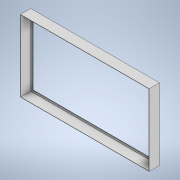
# Autodesk Inventor part: marco_ir
Saved by Autodesk Inventor 2021 (Build 250183000, 183)
## iProperties
Created: 2021-11-08
Part Number: marco_ir
Material: Genérico
Document SubType Name: Modeling
Designer: arthu
Density: 1 g/cm^3
Appearance: Valor por defecto
Author: arthu
Autodesk Inventor part; units mm, degrees
ref_plane "YZ Plane" through (0, 0, 0) normal (1, 0, 0) x (0, 1, 0)
ref_plane "XZ Plane" through (0, 0, 0) normal (0, 1, 0) x (-1, 0, 0)
ref_plane "XY Plane" through (0, 0, 0) normal (0, 0, 1) x (1, 0, 0)
sketch "Boceto1" plane through (0, 0, 0) normal (0, 0, 1) x (1, 0, 0)
  line L0 (260, -145) -> (-260, -145)
  line L1 (-260, -145) -> (-260, 145)
  line L2 (-260, 145) -> (260, 145)
  line L3 (260, 145) -> (260, -145)
  line L4 (260, -145) -> (-260, 145) construction
  line L5 (-260, -145) -> (260, 145) construction
  line L6 (250, -135) -> (-250, -135)
  line L7 (-250, -135) -> (-250, 135)
  line L8 (-250, 135) -> (250, 135)
  line L9 (250, 135) -> (250, -135)
  line L10 (250, -135) -> (-250, 135) construction
  line L11 (-250, -135) -> (250, 135) construction
  point P0 (0, 0)
  dimension "d0" = 520
  dimension "d1" = 290
  dimension "d2" = 500
  dimension "d3" = 270
  constraints: 24 end point, 4 midpoint, 4 parallel, 2 horizontal, 2 perpendicular
  measures "d0" distance of L1.end L2.end
  measures "d1" distance of L0.end L1.end
  measures "d2" distance of L7.end L8.end
  measures "d3" distance of L6.end L7.end
extrude "Extrusión1" add sketch "Boceto1" along normal blind 1.2
sketch "Boceto2" plane through (0, 0, 1.2) normal (0, 0, 1) x (1, 0, 0)
  line L0 (260, 145) -> (-260, 145) projected
  line L1 (-260, 145) -> (-260, -145) projected
  line L2 (260, -145) -> (260, 145) projected
  line L3 (-260, -145) -> (260, -145) projected
  line L4 (-258.8, 143.8) -> (258.8, 143.8)
  line L5 (258.8, 143.8) -> (258.8, -143.8)
  line L6 (258.8, -143.8) -> (-258.8, -143.8)
  line L7 (-258.8, -143.8) -> (-258.8, 143.8)
  point P0 (0, 0)
  dimension "d6" = 1.2
  constraints: 8 end point, 3 other
  measures "d6" distance between parallel lines of L0 L4
extrude "Extrusión2" add sketch "Boceto2" along normal blind 40
